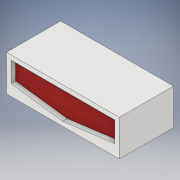
# Autodesk Inventor part: XGEN_LED-sidelooker_green
Saved by Autodesk Inventor 2019 (Build 230136000, 136)
## iProperties
Created: 2019-03-03
Part Number: XGEN_LED-sidelooker_green
Material: Generic
Document SubType Name: Modeling
Designer: Rene
Density: 1 g/cm^3
Appearance: White
Author: Rene
Autodesk Inventor part; units mm, degrees
ref_plane "YZ Plane" through (0, 0, 0) normal (1, 0, 0) x (0, 1, 0)
ref_plane "XZ Plane" through (0, 0, 0) normal (0, 1, 0) x (-1, 0, 0)
ref_plane "XY Plane" through (0, 0, 0) normal (0, 0, 1) x (1, 0, 0)
sketch "Sketch1" plane through (0, 0, 0) normal (0, 0, 1) x (1, 0, 0)
  line L0 (-1.25, 0) -> (1.25, 0)
  line L1 (1.25, 0) -> (1.25, 0.8)
  line L2 (1.25, 0.8) -> (-1.25, 0.8)
  line L3 (-1.25, 0.8) -> (-1.25, 0)
  point P0 (0, 0)
  dimension "d0" = 2.5
  dimension "d1" = 1.25
  dimension "d2" = 0.8
  constraints: 8 end point, 2 parallel, 1 horizontal, 1 perpendicular
  measures "d0" distance of L0.start L0.end
  measures "d1" distance of point (0, 0) L0.start
  measures "d2" distance of L2.end L0.start
extrude "Extrusion1" add sketch "Sketch1" along normal blind 1.2
sketch "Sketch2" plane through (0, 0, 1.2) normal (0, 0, 1) x (1, 0, 0)
  line L0 (-1.15, 0.7) -> (1.15, 0.7)
  line L1 (1.15, 0.7) -> (1.15, 0.25)
  line L2 (1.15, 0.25) -> (0, 0.1)
  line L3 (0, 0.1) -> (-1.15, 0.25)
  line L4 (-1.15, 0.25) -> (-1.15, 0.7)
  line L5 (-1.25, 0.8) -> (-1.25, 0) projected
  line L6 (1.25, 0) -> (1.25, 0.8) projected
  line L7 (1.25, 0.8) -> (-1.25, 0.8) projected
  point P0 (0, 0)
  dimension "d5" = 0.45
  dimension "d6" = 0.1
  dimension "d7" = 0.1
  dimension "d8" = 0.1
  dimension "d9" = 0.45
  dimension "d10" = 0.1
  constraints: 10 end point, 2 perpendicular, 1 horizontal
  measures "d5" distance of L3.end L0.start
  measures "d6" distance from line of L3.end L5
  measures "d7" distance from line of L6 L1.end
  measures "d8" distance between parallel lines of L7 L0
  measures "d9" distance of L0.end L1.end
  measures "d10" vertical distance of L2.end L5.end
extrude "Extrusion2" cut sketch "Sketch2" against normal blind 0.1
equation "\"d1\" = 0.5 * d0"
equation "\"d9\" = d5"
body "Solid1"
